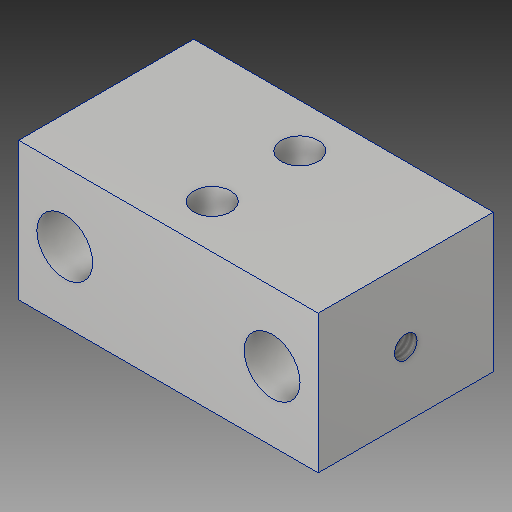
# Autodesk Inventor part: carro_boca_superior
Saved by Autodesk Inventor 2018 (Build 220112000, 112)
## iProperties
Created: 2018-05-17
Part Number: carro_boca_superior
Material: Alumínio 6061
Document SubType Name: Modeling
Designer: Usuario
Density: 2.7 g/cm^3
Appearance: Alumínio - Plano
Author: Usuario
Autodesk Inventor part; units mm, degrees
ref_plane "YZ Plane" through (0, 0, 0) normal (1, 0, 0) x (0, 1, 0)
ref_plane "XZ Plane" through (0, 0, 0) normal (0, 1, 0) x (-1, 0, 0)
ref_plane "XY Plane" through (0, 0, 0) normal (0, 0, 1) x (1, 0, 0)
sketch "Esboço1" plane through (0, 0, 0) normal (0, 0, 1) x (1, 0, 0)
  circle A0 centre (22.5, 0.8472) radius 5.995 construction
  circle A1 centre (-22.5, 0.8472) radius 5.995 construction
  line L0 (22.5, 0.8472) -> (32.5, 0.8472) construction
  line L1 (-22.5, 0.8472) -> (-32.5, 0.8472) construction
  line L2 (22.5, 0.8472) -> (-22.5, 0.8472) construction
  line L3 (-32.5, 15.8472) -> (32.5, 15.8472)
  line L4 (32.5, 15.8472) -> (32.5, -14.1528)
  line L5 (32.5, -14.1528) -> (-32.5, -14.1528)
  line L6 (-32.5, -14.1528) -> (-32.5, 15.8472)
  line L7 (-32.5, 15.8472) -> (32.5, -14.1528) construction
  line L8 (32.5, 15.8472) -> (-32.5, -14.1528) construction
  point P0 (0, 0)
  point P1 (0, 0.8472)
  dimension "d2" = 65
  dimension "d3" = 30
  constraints: 18 end point, 3 midpoint, 2 parallel, 1 collinear, 1 horizontal, 1 perpendicular, 1 point on line
  measures "d2" distance of L4.end L5.end
  measures "d3" distance of L3.end L4.end
extrude "Extrusão1" add sketch "Esboço1" along normal blind 38
sketch "Esboço2" plane through (0, 0, 38) normal (0, 0, 1) x (1, 0, 0)
  circle A0 centre (22.5, 0.8472) radius 5.995 construction
  circle A1 centre (-22.5, 0.8472) radius 5.995 construction
  point P0 (0, 0)
hole "Furo1" at (-22.5, 0.8472, 38) at (22.5, 0.8472, 38) direction (0, 0, -1) diameter 12.1 end through all
sketch "Esboço3" plane through (32.5, -14.1528, 0) normal (1, 0, 0) x (0, 0, -1)
  line L0 (0, 30) -> (-38, 30) construction
  line L1 (-19, 30) -> (-19, 0) construction
  line L2 (0, 0) -> (-38, 0) construction
  line L3 (-19, 14.1528) -> (0, 14.1528) construction
  constraints: 4 end point, 2 midpoint, 1 horizontal, 1 point on line
hole "Furo2" at (32.5, 0, 19) direction (-1, 0, 0) diameter 4.917 end up to face face through (22.5, 0.8472, -43.0494) facing (0, 0, 1) round with radius 6.05 far side yes thread size "M6x1" class "6H" standard "ANSI Metric M Profile"
sketch "Esboço4" plane through (-32.5, -14.1528, 0) normal (0, -1, 0) x (1, 0, 0)
  line L0 (65, 0) -> (65, 38) projected
  line L1 (65, 19) -> (0, 19) construction
  line L2 (0, 0) -> (0, 38) projected
  line L3 (0, 38) -> (65, 38) projected
  line L4 (32.5, 19) -> (32.5, 28.5) construction
  line L5 (32.5, 19) -> (32.5, 9.5) construction
  point P0 (32.5, 0)
  dimension "d20" = 9.5
  dimension "d21" = 9.5
  constraints: 6 end point, 2 midpoint
  measures "d20" distance of L4.start L4.end
  measures "d21" distance of L4.start L5.end
hole "Furo3" at (0, -14.1528, 28.5) at (0, -14.1528, 9.5) direction (0, 1, 0) diameter 8 end through all counterbore diameter 14 counterbore depth 16
